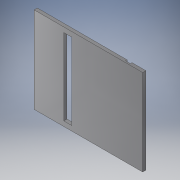
# Autodesk Inventor part: baseplate
Saved by Autodesk Inventor 2019 (Build 230136000, 136)
## iProperties
Created: 2018-10-03
Part Number: baseplate
Material: Aluminum 6061-AHC
Document SubType Name: Modeling
Designer: LillaHunden
Density: 2.7 g/cm^3
Appearance: Aluminum - Dark
Mass: 2025 g
Surface Area: 1610 cm^2
Volume: 750 cm^3
Author: LillaHunden
Autodesk Inventor part; units mm, degrees
ref_plane "YZ Plane" through (0, 0, 0) normal (1, 0, 0) x (0, 1, 0)
ref_plane "XZ Plane" through (0, 0, 0) normal (0, 1, 0) x (-1, 0, 0)
ref_plane "XY Plane" through (0, 0, 0) normal (0, 0, 1) x (1, 0, 0)
sketch "Sketch1" plane through (0, 0, 0) normal (0, 0, 1) x (1, 0, 0)
  line L0 (-216.6526, -262.3711) -> (123.3474, -262.3711)
  line L1 (123.3474, -262.3711) -> (123.3474, 7.6289)
  line L2 (123.3474, 7.6289) -> (-216.6526, 7.6289)
  line L3 (-216.6526, 7.6289) -> (-216.6526, -262.3711)
  point P0 (0, 0)
  dimension "d0" = 340
  dimension "d1" = 270
  constraints: 8 end point, 2 parallel, 1 horizontal, 1 perpendicular
  measures "d0" distance of L2.end L1.end
  measures "d1" distance of L1.end L0.end
extrude "Extrusion1" add sketch "Sketch1" along normal blind 10
sketch "Sketch2" plane through (0, 0, 0) normal (0, 0, -1) x (-1, 0, 0)
  line L0 (-66.3474, -50.3711) -> (-66.3474, -52.3711) construction
  line L1 (-66.3474, -52.3711) -> (-47.3474, -52.3711) construction
  line L2 (-47.3474, -52.3711) -> (-47.3474, -37.3711) construction
  line L3 (-47.3474, -37.3711) -> (-64.7974, -37.3711) construction
  line L4 (-64.7974, -37.3711) -> (-64.7974, -42.3711) construction
  line L5 (-64.7974, -42.3711) -> (-79.8974, -42.3711) construction
  line L6 (-79.8974, -42.3711) -> (-79.8974, -37.3711) construction
  line L7 (-79.8974, -37.3711) -> (-97.3474, -37.3711) construction
  line L8 (-97.3474, -37.3711) -> (-97.3474, -52.3711) construction
  line L9 (-97.3474, -52.3711) -> (-78.3474, -52.3711) construction
  line L10 (-78.3474, -52.3711) -> (-78.3474, -50.3711) construction
  line L11 (-78.3474, -50.3711) -> (-66.3474, -50.3711) construction
  line L12 (-79.7974, -42.3711) -> (-79.7974, -9.1428) construction
  line L13 (-64.7974, -42.3711) -> (-79.7974, -42.3711) construction
  line L14 (-64.7974, -42.3711) -> (-64.7974, -9.1428) construction
  line L15 (-79.7974, -26.2239) -> (-79.7974, -29.3711) construction
  line L16 (-79.7974, -29.3711) -> (-64.7974, -29.3711) construction
  line L17 (-64.7974, -29.3711) -> (-64.7974, -26.2239) construction
  line L18 (-64.7974, -26.2239) -> (-79.7974, -26.2239) construction
  line L19 (-79.7974, 7.2343) -> (-64.7974, 7.2343) construction
  line L20 (-79.7974, -9.1428) -> (-79.7974, 7.2343) construction
  line L21 (-64.7974, 7.2343) -> (-64.7974, -9.1428) construction
  line L22 (-123.3474, 7.6289) -> (216.6526, 7.6289) projected
  line L23 (-79.9974, 7.6289) -> (-79.9974, -37.1711)
  line L24 (-79.9974, -37.1711) -> (-97.5474, -37.1711)
  line L25 (-97.5474, -37.1711) -> (-97.5474, -52.5711)
  line L26 (-97.5474, -52.5711) -> (-47.1474, -52.5711)
  line L27 (-47.1474, -52.5711) -> (-47.1474, -37.1711)
  line L28 (-47.1474, -37.1711) -> (-64.5974, -37.1711)
  line L29 (-64.5974, -37.1711) -> (-64.5974, 7.6289)
  line L30 (-79.9974, 7.6289) -> (-64.5974, 7.6289)
  circle A0 centre (-57.3474, -44.8711) radius 1.621 projected
  circle A1 centre (-87.3474, -44.8711) radius 1.621 projected
  line L31 (-64.7974, -9.1428) -> (-79.7974, -9.1428) projected
  line L32 (-64.7974, -9.1428) -> (-79.7974, -9.1428) projected
  circle A2 centre (-72.2869, -16.8711) radius 1.621 projected
  circle A3 centre (-72.2869, -36.8711) radius 1.621 projected
  point P0 (0, 0)
  dimension "d4" = 0.2
  dimension "d5" = 0.2
  dimension "d6" = 0.2
  dimension "d7" = 0.2
  dimension "d8" = 0.2
  dimension "d9" = 0.2
  constraints: 16 end point, 7 perpendicular, 4 point on line
  measures "d4" distance between parallel lines of L14 L29
  measures "d5" distance between parallel lines of L3 L28
  measures "d6" distance between parallel lines of L2 L27
  measures "d7" distance between parallel lines of L1 L26
  measures "d8" distance between parallel lines of L8 L25
  measures "d9" distance between parallel lines of L12 L23
extrude "Extrusion2" cut sketch "Sketch2" against normal blind 5 contours L22 L29 L28 L27 L26 L25 L24 L23 | A0 | A1 | A2 | A3
body "Solid1"
